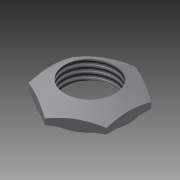
# Autodesk Inventor part: 13_8
Saved by Autodesk Inventor 2015 (Build 190159000, 159)
## iProperties
Created: 2015-04-01
Part Number: 13_8
Material: Generic
Document SubType Name: Modeling
Designer: WASHHSST
Density: 1 g/cm^3
Appearance: Default
Author: WASHHSST
Autodesk Inventor part; units mm, degrees
ref_plane "YZ Plane" through (0, 0, 0) normal (1, 0, 0) x (0, 1, 0)
ref_plane "XZ Plane" through (0, 0, 0) normal (0, 1, 0) x (-1, 0, 0)
sketch "Sketch1" plane through (0, 0, 0) normal (0, 1, 0) x (-1, 0, 0)
  circle A0 centre (0, 0) radius 9.9187
  line L0 (9.9187, -5.7266) -> (0, -11.4531)
  line L1 (0, -11.4531) -> (-9.9187, -5.7266)
  line L2 (-9.9187, -5.7266) -> (-9.9187, 5.7266)
  line L3 (-9.9187, 5.7266) -> (0, 11.4531)
  line L4 (0, 11.4531) -> (9.9187, 5.7266)
  line L5 (9.9187, 5.7266) -> (9.9187, -5.7266)
  line L6 (0, 13.376) -> (0, -12.9473) construction
  point P0 (9.9187, 0)
  dimension "d0" = 19.8374
  constraints: 14 end point, 2 coincident, 1 horizontal alignment, 1 midpoint, 1 parallel, 1 vertical, 15 other
extrude "Extrusion1" add sketch "Sketch1" along normal blind 4.3688
sketch "Sketch2" plane through (0, 0, 0) normal (0, -1, 0) x (1, 0, 0)
  circle A0 centre (0, 0) radius 9.9187
  line L0 (0, 11.4531) -> (9.9187, 5.7266) projected
  constraints: 1 centre point, 1 coincident, 1 tangent
extrude "Extrusion2" add sketch "Sketch2" along normal blind 0.4064
sketch "Sketch3" plane through (0, 4.3688, 0) normal (0, 1, 0) x (1, 0, 0)
  point P0 (0, 0)
  point P1 (0, 0)
  constraints: 1 coincident
hole "Hole1" at (0, 4.3688, 0) direction (0, -1, 0) diameter 12.7508 end through all
thread "Thread1" size "9/16-18 UNF" class "2B" standard "ANSI Unified Screw Threads" full length
ref_plane "Work Plane1" through (0, 0, -5.7266) normal (1, 0, 0) x (0, 0, -1)
sketch "Sketch5" plane through (0, 0, -5.7266) normal (1, 0, 0) x (0, 0, -1)
  line L0 (-12.102, 4.3688) -> (0.6488, 4.3688) projected
  line L1 (-12.102, 4.3688) -> (-17.1797, 4.3688)
  line L2 (-12.102, 4.3688) -> (-17.1797, 1.4372)
  line L3 (-17.1797, 1.4372) -> (-17.1797, 4.3688)
  line L4 (-5.7266, 0) -> (-5.7266, 18.228)
  dimension "d17" = 30
  constraints: 9 end point, 2 vertical, 1 horizontal
  measures "d17" angle of L1 L2
revolve "Revolution1" cut sketch "Sketch5" angle 360 about axis through (0, 0, 0) along (0, 1, 0)
body "Solid1"
